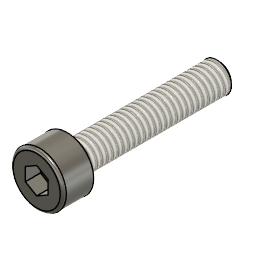
_2CWA9TJD5Y5ZICN82B6K2HIVUen-US11.b4c415c8-f10c-463e-afa1-e01077a5fb48 (Autodesk Fusion 360 design; units mm, degrees)
description: Forged Hexagon Socket Head Cap Screw ANSI B18.3.1M - M4x0.7 x 20
part number: FSHCS ANSI B18.3.1M - M4x0.7 x 20 Steel Grade 2 Plain
Autodesk Fusion 360 part; units mm, degrees
sketch "Sketch1" plane through (0, 0, 0) normal (0, 1, 0) x (1, 0, 0)
  line L0 (-2, 0) -> (-2, 20)
  line L1 (-2, 20) -> (0, 20)
  line L2 (0, 20) -> (0, -4)
  line L3 (-2, 0) -> (-3.5, 0)
  line L4 (-3.5, 0) -> (-3.5, -4)
  line L5 (-3.5, -4) -> (0, -4)
  dimension "d101" = 20
  dimension "d102" = 4
  dimension "d109" = 7
  dimension "d110" = 4
  constraint perpendicular L0 L1
  constraint collinear origin L1.end L2.end
  constraint perpendicular L0 L3
  constraint coincident origin L3
  constraint vertical L2
  constraint coincident L2 L5.end
  constraint perpendicular L2 L5
  measures "d101" distance of origin L1
  measures "d102" distance of L3.end L5
revolve "Revolve1" add sketch "Sketch1" angle 360 about axis through (0, 0, -20) along (0, 0, 1)
ref_plane "WorkPlane1" through (0, 0, 4) normal (0, 0, 1) x (1, 0, 0)
sketch "Sketch6" plane through (0, 0, 4) normal (0, 0, 1) x (1, 0, 0)
  line L0 (0, -1.7321) -> (1.5, -0.866)
  line L1 (1.5, -0.866) -> (1.5, 0.866)
  line L2 (1.5, 0.866) -> (0, 1.7321)
  line L3 (0, 1.7321) -> (-1.5, 0.866)
  line L4 (-1.5, 0.866) -> (-1.5, -0.866)
  line L5 (-1.5, -0.866) -> (0, -1.7321)
  dimension "d111" = 3
  constraint vertical L1
  measures "d111" distance of L1 L4
extrude "Extrude1" cut sketch "Sketch6" against normal blind 2
extrude "Extrude2" cut 1 faces at (-0.5, -0.2887, 2) along direction (0, 0, -1) blind 2 draft -85
thread "Thread3" "ANSI Metric M Profile 4.0 M4x0.7 M4x0.7 4g6g" major diameter 3.908 minor diameter 3.128 pitch 0.7 angle 60 resizes the face on face at (-1.9975, 0.0997, -13.3333) from (0, 0, -1.2588) to (0, 0, -20)
fillet "Fillet4" radius 0.4 1 edges at (-3.2631, 1.2657, 4)
sketch "Sketch7" plane through (0, 0, 0) normal (0, 1, 0) x (1, 0, 0)
  line L0 (-2.04, 20) -> (-2.04, 19.5706)
  line L1 (-2.04, 19.5706) -> (-1.5706, 20)
  line L2 (0, 20) -> (0, -4)
  line L3 (-2.04, 20) -> (0, 20)
  dimension "d104" = 1.5706
  dimension "d105" = 2.04
  dimension "d106" = 0.4294
  constraint coincident L2.start L3.end
  constraint perpendicular L2 L3
  constraint coincident L1.end L3
  constraint perpendicular L0 L3
  measures "d104" distance of L1.end L2
  measures "d105" distance of L0 L2.start
  measures "d106" distance of L0.end L3
revolve "Revolve3" cut sketch "Sketch7" angle 360 about axis through (0, 0, 1.75) along (0, 0, 1)
equation "adsk_nomlen = 20.00 mm"
equation "adsk_headh = 4.00 mm"
equation "adsk_headdia = 7.00 mm"
equation "adsk_nomdia = 4.00 mm"
equation "adsk_philwidth = 3.00 mm"
equation "d31 = -adsk_phildepth"
equation "adsk_phildepth = 2.00 mm"
equation "d71 = adsk_headh"
equation "d76 = -adsk_phildepth"
equation "adsk_thrlen = 18.74117 mm"
equation "d86 = adsk_nomdia * 0.1"
equation "adsk_startlen = 0.429415 mm"
equation "adsk_endpointdia = 3.14117 mm"
equation "d101 = adsk_nomlen"
equation "d102 = adsk_headh"
equation "d104 = adsk_endpointdia / 2"
equation "d105 = adsk_nomdia * 0.51"
equation "d106 = adsk_startlen"
equation "d108 = min(adsk_thrlen; adsk_nomlen - 0.001 mm)"
equation "d109 = adsk_headdia"
equation "d110 = adsk_nomdia"
equation "d111 = adsk_philwidth"
